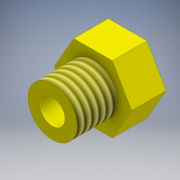
# Autodesk Inventor part: Premistoppa
Saved by Autodesk Inventor 2016 (Build 200138000, 138)
## iProperties
Created: 2016-09-09
Part Number: Premistoppa
Material: Generic
Document SubType Name: Modeling
Designer: Muhammad
Density: 1 g/cm^3
Appearance: Default
Author: Muhammad
Autodesk Inventor part; units mm, degrees
ref_plane "YZ Plane" through (0, 0, 0) normal (1, 0, 0) x (0, 1, 0)
ref_plane "XZ Plane" through (0, 0, 0) normal (0, 1, 0) x (-1, 0, 0)
ref_plane "XY Plane" through (0, 0, 0) normal (0, 0, 1) x (1, 0, 0)
sketch "Sketch1" plane through (0, 0, 0) normal (0, 1, 0) x (-1, 0, 0)
  line L0 (-9.5, 0) -> (-4.75, 8.2272)
  line L1 (-4.75, 8.2272) -> (4.75, 8.2272)
  line L2 (4.75, 8.2272) -> (9.5, 0)
  line L3 (9.5, 0) -> (4.75, -8.2272)
  line L4 (4.75, -8.2272) -> (-4.75, -8.2272)
  line L5 (-4.75, -8.2272) -> (-9.5, 0)
  point P0 (0, 0)
  point P1 (0, 0)
  dimension "d2" = 9.5
  constraints: 12 end point, 1 coincident, 13 other
  measures "d2" distance of point (0, 0) L0.start
extrude "Extrusion1" add sketch "Sketch1" along normal blind 8.5
sketch "Sketch2" plane through (0, 0, 0) normal (0, -1, 0) x (1, 0, 0)
  circle A0 centre (0, 0) radius 6
  circle A1 centre (0, 0) radius 3.1
  dimension "d5" = 12
  dimension "d6" = 6.2
  constraints: 2 centre point, 2 coincident
  measures "d5" diameter of A0
  measures "d6" diameter of A1
extrude "Extrusion2" add sketch "Sketch2" along normal blind 10
sketch "Sketch3" plane through (0, 0, 0) normal (0, -1, 0) x (1, 0, 0)
  circle A0 centre (0, 0) radius 3.1
  constraints: 1 centre point, 1 coincident
extrude "Extrusion3" cut sketch "Sketch3" against normal through all
thread "Thread1" size "M12x1.75" class "6g" standard "ANSI Metric M Profile" full length
body "Solid1"
